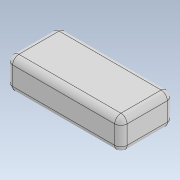
# Autodesk Inventor part: BatteryV1
Saved by Autodesk Inventor 2020.2 (Build 242310000, 310)
## iProperties
Created: 2020-04-30
Part Number: BatteryV1
Material: Generic
Document SubType Name: Modeling
Designer: Haashim Rehan
Density: 1 g/cm^3
Appearance: Default
Author: Haashim Rehan
Autodesk Inventor part; units mm, degrees
ref_plane "YZ Plane" through (0, 0, 0) normal (1, 0, 0) x (0, 1, 0)
ref_plane "XZ Plane" through (0, 0, 0) normal (0, 1, 0) x (-1, 0, 0)
ref_plane "XY Plane" through (0, 0, 0) normal (0, 0, 1) x (1, 0, 0)
sketch "Sketch1" plane through (0, 0, 0) normal (0, 0, 1) x (1, 0, 0)
  line L0 (-37, -10) -> (37, -10)
  line L1 (37, -10) -> (37, 10)
  line L2 (37, 10) -> (-37, 10)
  line L3 (-37, 10) -> (-37, -10)
  line L4 (-37, -10) -> (37, 10) construction
  line L5 (37, -10) -> (-37, 10) construction
  point P0 (0, 0)
  dimension "d0" = 74
  dimension "d1" = 20
  constraints: 12 end point, 2 midpoint, 2 parallel, 1 horizontal, 1 perpendicular
  measures "d0" distance of L2.end L1.end
  measures "d1" distance of L1.end L0.end
extrude "Extrusion1" add sketch "Sketch1" along normal mid plane 34
fillet "Fillet1" radius 4 12 edges at (37, 0, 17) (37, 10, 0) (0, 10, 17) (-37, 10, 0) (-37, 0, 17) (-37, -10, 0) (0, -10, 17) (37, -10, 0) (0, 10, -17) (-37, 0, -17) (0, -10, -17) (37, 0, -17)
body "Solid1"
